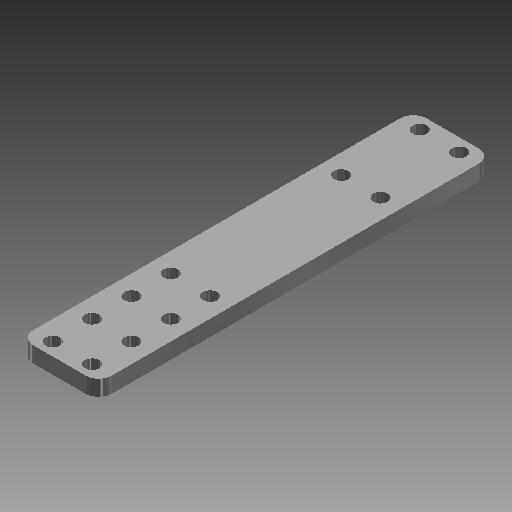
# Autodesk Inventor part: GARFO
Saved by Autodesk Inventor 2017 (Build 210142000, 142)
## iProperties
Created: 2016-08-09
Part Number: GARFO
Material: Aluminium AW-7020
Document SubType Name: Modeling
Designer: EriveltonDell
Density: 2.78 g/cm^3
Appearance: Stainless - Brushed
Mass: 1234.07 g
Surface Area: 731.335 cm^2
Volume: 443.911 cm^3
Author: EriveltonDell
Autodesk Inventor part; units mm, degrees
ref_plane "YZ Plane" through (0, 0, 0) normal (1, 0, 0) x (0, 1, 0)
ref_plane "XZ Plane" through (0, 0, 0) normal (0, 1, 0) x (-1, 0, 0)
ref_plane "XY Plane" through (0, 0, 0) normal (0, 0, 1) x (1, 0, 0)
sketch "Sketch7" plane through (0, 0, 0) normal (0, 1, 0) x (-1, 0, 0)
  line L0 (5, 0) -> (25, 0)
  line L1 (30, 5) -> (30, 150)
  line L2 (25, 150) -> (5, 150)
  line L3 (0, 145) -> (0, 5)
  line L4 (30, 145) -> (30, 145)
  line L5 (30, 145) -> (22.5, 145)
  circle A0 centre (22.5, 145) radius 2.75
  circle A1 centre (22.5, 130) radius 2.75
  circle A2 centre (7.5, 145) radius 2.75
  circle A3 centre (7.5, 130) radius 2.75
  line L6 (22.5, 130) -> (30, 130)
  line L7 (30, 130) -> (30, 125)
  circle A4 centre (22.5, 35) radius 2.75
  circle A5 centre (22.5, 5) radius 2.75
  circle A6 centre (7.5, 35) radius 2.75
  circle A7 centre (7.5, 5) radius 2.75
  circle A8 centre (22.5, 115) radius 2.75
  circle A9 centre (7.5, 115) radius 2.75
  circle A10 centre (22.5, 100) radius 2.75
  circle A11 centre (7.5, 100) radius 2.75
  arc A12 (30, 145) -> (25, 150) centre (25, 145) ccw
  arc A13 (5, 150) -> (0, 145) centre (5, 145) ccw
  arc A14 (25, 0) -> (30, 5) centre (25, 5) ccw
  arc A15 (0, 5) -> (5, 0) centre (5, 5) ccw
  point P0 (0, 0)
  point P1 (30, 0)
  point P2 (0, 150)
  dimension "d141" = 30
  dimension "d142" = 150
  dimension "d143" = 5
  dimension "d144" = 7.5
  dimension "d145" = 5.5
  dimension "d148" = 15
  dimension "d151" = 15
  dimension "d154" = 5
  dimension "d159" = 5.5
  dimension "d160" = 30
  dimension "d161" = 15
  dimension "d162" = 5
  constraints: 16 centre point, 16 end point, 11 point on line, 8 point on circle, 8 tangent, 3 equal radius, 3 perpendicular, 2 horizontal, 2 parallel, 1 coincident, 1 vertical, 14 other
  measures "d141" distance of point (0, 150) L1.end
  measures "d142" distance of L1.end point (30, 0)
  measures "d143" distance of L1.end L4.end
  measures "d144" distance of L4.end L5.end
  measures "d145" diameter of A0
  measures "d148" distance of A0.centre L6.start
  measures "d151" distance of A0.centre A2.centre
  measures "d154" distance of L6.end L7.end
  measures "d159" diameter of A4
  measures "d160" distance of A4.centre A5.centre
  measures "d161" distance of A4.centre A6.centre
  measures "d162" radius of A12
extrude "Extrusion5" add sketch "Sketch7" along normal blind 6
body "Solid4"
